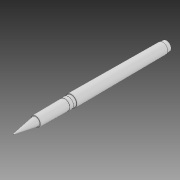
# Autodesk Inventor part: pen
Saved by Autodesk Inventor 2020 (Build 240168000, 168)
## iProperties
Created: 2020-07-24
Part Number: pen
Material: Generic
Document SubType Name: Modeling
Designer: DDeGo
Density: 1 g/cm^3
Appearance: Default
Author: DDeGo
Autodesk Inventor part; units mm, degrees
ref_plane "YZ Plane" through (0, 0, 0) normal (1, 0, 0) x (0, 1, 0)
ref_plane "XZ Plane" through (0, 0, 0) normal (0, 1, 0) x (-1, 0, 0)
ref_plane "XY Plane" through (0, 0, 0) normal (0, 0, 1) x (1, 0, 0)
sketch "Sketch1" plane through (0, 0, 0) normal (1, 0, 0) x (0, 1, 0)
  line L0 (0, 0) -> (3.875, 0)
  line L1 (3.875, 0) -> (3.875, 3.2)
  line L2 (3.875, 3.2) -> (4.25, 3.2)
  line L3 (4.25, 3.2) -> (4.8, 80.3)
  line L4 (4.8, 80.3) -> (4.325, 80.3)
  line L5 (0, 0) -> (0, 129.1)
  line L6 (4.325, 80.3) -> (4.325, 82.8)
  line L7 (4.325, 82.8) -> (4.4, 82.8)
  line L8 (4.4, 82.8) -> (4.4, 85.8)
  line L9 (4.4, 85.8) -> (4.25, 85.8)
  line L10 (4.25, 85.8) -> (4, 110.3)
  line L11 (4, 110.3) -> (3.375, 110.3)
  line L12 (3.375, 110.3) -> (0.2, 129.1)
  line L13 (0.2, 129.1) -> (0, 129.1)
  dimension "d0" = 3.875
  dimension "d1" = 3.2
  dimension "d2" = 4.25
  dimension "d3" = 4.8
  dimension "d4" = 80.3
  dimension "d5" = 4.325
  dimension "d6" = 2.5
  dimension "d7" = 3
  dimension "d8" = 4.4
  dimension "d9" = 4.25
  dimension "d10" = 4
  dimension "d11" = 3.375
  dimension "d12" = 129.1
  dimension "d13" = 30
  dimension "d15" = 0.2
  constraints: 28 end point, 6 perpendicular, 3 horizontal, 2 vertical
  measures "d0" distance between parallel lines of L5 L1
  measures "d1" distance of L0.end L1.end
  measures "d2" distance from line of L5 L2.end
  measures "d3" distance from line of L5 L3.end
  measures "d4" distance between parallel lines of L0 L4
  measures "d5" distance from line of L5 L4.end
  measures "d6" distance of L4.end L6.end
  measures "d7" distance of L7.end L8.end
  measures "d8" distance between parallel lines of L5 L8
  measures "d9" distance from line of L5 L9.end
  measures "d10" distance from line of L5 L10.end
  measures "d11" distance from line of L5 L11.end
  measures "d12" distance of L0.start L5.end
  measures "d13" distance between parallel lines of L4 L11
  measures "d15" distance of L12.end L5.end
revolve "Revolution1" add sketch "Sketch1" angle 360 about axis through (0, 0, 0) along (0, 0, 1)
body "Solid1"
